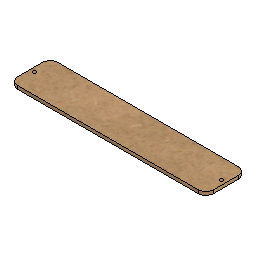
Leds nivel accidente capa3 (Autodesk Fusion 360 design; units mm, degrees)
Autodesk Fusion 360 part; units mm, degrees
sketch "Sketch1" plane through (0, 0, 0) normal (0, 0, 1) x (1, 0, 0)
  line L0 (-81, 18) -> (81, 18)
  line L1 (88, 11) -> (88, -11)
  line L2 (81, -18) -> (-81, -18)
  line L3 (-88, -11) -> (-88, 11)
  line L4 (-88, 18) -> (88, -18) construction
  line L5 (88, 18) -> (-88, -18) construction
  arc A0 (-81, 18) -> (-88, 11) centre (-81, 11) ccw
  arc A1 (-88, -11) -> (-81, -18) centre (-81, -11) ccw
  arc A2 (81, -18) -> (88, -11) centre (81, -11) ccw
  arc A3 (88, 11) -> (81, 18) centre (81, 11) ccw
  line L6 (0, 0) -> (27, 0) construction
  circle A4 centre (-84, 0) radius 1.5
  line L7 (0, 0) -> (0, 18) construction
  circle A5 centre (84, 0) radius 1.5
  dimension "d28" = 176
  dimension "d29" = 36
  dimension "d30" = 7
  dimension "d35" = 3
  dimension "d36" = 4
  dimension "d37" = 18
  constraint coincident L6.start L7.start
  constraint perpendicular L0 L1
  constraint parallel L0 L2
  constraint parallel L1 L3
  constraint horizontal L0
  constraint coincident L4 L6.start
  constraint coincident L5 L6.start
  constraint coincident L4.start L0
  constraint coincident L4.start L3
  constraint tangent L0 A0
  constraint tangent L3 A0
  constraint coincident L5.end L3
  constraint coincident L5.end L2
  constraint tangent L3 A1
  constraint tangent L2 A1
  constraint equal A0 A1
  constraint coincident L4.end L2
  constraint coincident L4.end L1
  constraint tangent L2 A2
  constraint tangent L1 A2
  constraint equal A0 A2
  constraint coincident L5.start L1
  constraint coincident L5.start L0
  constraint tangent L1 A3
  constraint tangent L0 A3
  constraint equal A0 A3
  constraint midpoint L0 L7.end
  constraint symmetric A4 L7 A5
  measures "d28" distance of L4.end L5.end
  measures "d29" distance of L5.start L4.end
  measures "d30" radius of A0
  measures "d35" diameter of A4
  measures "d36" distance of L3 A4.centre
  measures "d37" distance of L0 A4.centre
extrude "Extrude7" add sketch "Sketch1" along normal blind 3
sketch "Sketch3" plane through (0, 0, 3) normal (0, 0, 1) x (-1, 0, 0)
  circle A0 centre (0, -13) radius 1.5
  circle A1 centre (-85, 0) radius 1.5
  circle A2 centre (0, 13) radius 1.5
  circle A3 centre (85, 0) radius 1.5
  line L0 (-79, 9) -> (79, 9)
  line L1 (79, 9) -> (79, -9)
  line L2 (79, -9) -> (-79, -9)
  line L3 (-79, -9) -> (-79, 9)
  arc A4 (-83, 18) -> (-90, 11) centre (-83, 11) ccw
  line L4 (-90, 11) -> (-90, -11)
  arc A5 (-90, -11) -> (-83, -18) centre (-83, -11) ccw
  line L5 (-83, -18) -> (83, -18)
  arc A6 (83, -18) -> (90, -11) centre (83, -11) ccw
  line L6 (90, -11) -> (90, 11)
  arc A7 (90, 11) -> (83, 18) centre (83, 11) ccw
  line L7 (83, 18) -> (-83, 18)
  circle A8 centre (0, 13) radius 1.5
